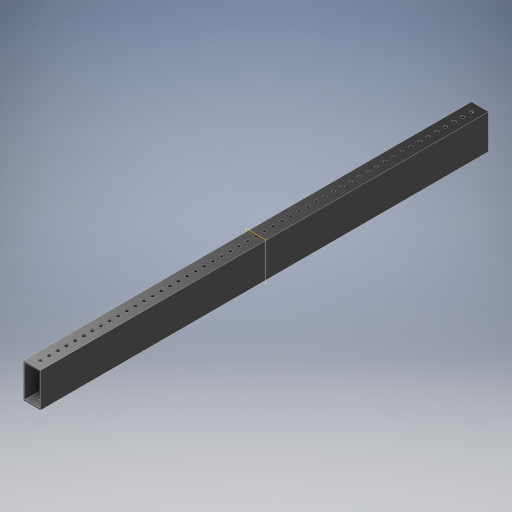
# Autodesk Inventor part: 2024-100-001-Left-Right-Extrusions
Saved by Autodesk Inventor 2024.2 (Build 282272000, 272)
## iProperties
RuleStatus: InUse
Created: 2024-01-06
Part Number: 2024-100-001-Left-Right-Extrusions
Material: Aluminum 6061
Document SubType Name: Modeling
Designer: rohan
Density: 2.7 g/cm^3
Appearance: Glossy - Black
AfterDocNew0: OnNew
AfterDocNew1: Configure
AfterAnyParamChange0: Run All Loop
AfterAnyUserParamChange0: Run All Loop
AfterFeatureSuppressionChange0: Run All Loop
PartBodyChanged0: Run All Loop
Author: rohan
Autodesk Inventor part; units mm, degrees
ref_plane "YZ Plane" through (0, 0, 0) normal (1, 0, 0) x (0, 1, 0)
sketch "Corner" plane through (0, 0, 0) normal (0, 0, 1) x (1, 0, 0)
  line L0 (-6.5971, 24.384) -> (-10.9924, 24.384)
  arc A0 (-10.9924, 24.384) -> (-11.684, 23.6924) centre (-10.9924, 23.6924) ccw
  line L1 (-11.684, 23.6924) -> (-11.684, 19.2971)
  arc A1 (-11.684, 19.2971) -> (-10.3994, 18.9412) centre (-10.9924, 19.2971) ccw
  arc A2 (-6.2412, 23.0994) -> (-6.5971, 24.384) centre (-6.5971, 23.6924) ccw
  arc A3 (-6.2412, 23.0994) -> (-10.3994, 18.9412) centre (0, 12.7) ccw
  arc A4 (-4.8895, 22.679) -> (-9.979, 17.5895) centre (0, 12.7) ccw
  line L2 (-9.979, 17.5895) -> (-11.684, 17.5895)
  line L3 (-4.8895, 22.679) -> (-4.8895, 24.384)
  line L4 (-11.684, 23.6924) -> (-11.684, 24.384)
  line L5 (-11.684, 24.384) -> (-10.9924, 24.384)
  line L6 (-11.684, 17.5895) -> (-11.684, 19.2971)
  line L7 (-4.8895, 24.384) -> (-6.5971, 24.384)
  point P0 (-8.4584, 21.1584)
  dimension "d3" = 1.5875
  dimension "d4" = 11.1125
  dimension "d8" = 0
  dimension "d9" = 0
  dimension "d10" = 0
  dimension "d11" = 2.159
  dimension "d12" = 2.159
  dimension "d5" = 1.016
  dimension "d6" = 1.705
  dimension "d7" = 0.6916
  measures "d6" distance of point (-4.889, 22.679) L7.start
  measures "d7" radius of A0
sketch "MAXTube" plane through (0, 0, 0) normal (0, 0, 1) x (1, 0, 0)
  arc A0 (-5.3052, 13.2526) -> (-8.8244, 11.2207) centre (0, 0) ccw
  arc A1 (-11.1818, 11.0863) -> (-8.8244, 11.2207) centre (-10.0994, 12.842) ccw
  arc A2 (-11.1818, 11.0863) -> (-13.8706, 10.5882) centre (-12.251, 9.3519) ccw
  arc A3 (-13.8706, 10.5882) -> (-16.1049, 6.7182) centre (0, 0) ccw
  arc A4 (-16.1049, 6.7182) -> (-15.1919, 4.1406) centre (-14.2245, 5.9338) ccw
  arc A5 (-14.1297, 2.0318) -> (-15.1919, 4.1406) centre (-16.1712, 2.3254) ccw
  arc A6 (-14.1297, 2.0318) -> (-14.1297, -2.0318) centre (0, 0) ccw
  arc A7 (-15.1919, -4.1406) -> (-14.1297, -2.0318) centre (-16.1712, -2.3254) ccw
  arc A8 (-15.1919, -4.1406) -> (-16.1049, -6.7182) centre (-14.2245, -5.9338) ccw
  arc A9 (-16.1049, -6.7182) -> (-13.8706, -10.5882) centre (0, 0) ccw
  arc A10 (-13.8706, -10.5882) -> (-11.1818, -11.0863) centre (-12.251, -9.3519) ccw
  arc A11 (-8.8244, -11.2207) -> (-11.1818, -11.0863) centre (-10.0994, -12.842) ccw
  arc A12 (-8.8244, -11.2207) -> (-5.3052, -13.2526) centre (0, 0) ccw
  arc A13 (-4.0101, -15.2268) -> (-5.3052, -13.2526) centre (-6.0718, -15.1673) ccw
  arc A14 (-4.0101, -15.2268) -> (-2.2343, -17.3064) centre (-1.9735, -15.2856) ccw
  arc A15 (-2.2343, -17.3064) -> (2.2343, -17.3064) centre (0, 0) ccw
  arc A16 (2.2343, -17.3064) -> (4.0101, -15.2268) centre (1.9735, -15.2856) ccw
  arc A17 (5.3052, -13.2526) -> (4.0101, -15.2268) centre (6.0718, -15.1673) ccw
  arc A18 (5.3052, -13.2526) -> (8.8244, -11.2207) centre (0, 0) ccw
  arc A19 (11.1818, -11.0863) -> (8.8244, -11.2207) centre (10.0994, -12.842) ccw
  arc A20 (11.1818, -11.0863) -> (13.8706, -10.5882) centre (12.251, -9.3519) ccw
  arc A21 (13.8706, -10.5882) -> (16.1049, -6.7182) centre (0, 0) ccw
  arc A22 (16.1049, -6.7182) -> (15.1919, -4.1406) centre (14.2245, -5.9338) ccw
  arc A23 (14.1297, -2.0318) -> (15.1919, -4.1406) centre (16.1712, -2.3254) ccw
  arc A24 (14.1297, -2.0318) -> (14.1297, 2.0318) centre (0, 0) ccw
  arc A25 (15.1919, 4.1406) -> (14.1297, 2.0318) centre (16.1712, 2.3254) ccw
  arc A26 (15.1919, 4.1406) -> (16.1049, 6.7182) centre (14.2245, 5.9338) ccw
  arc A27 (16.1049, 6.7182) -> (13.8706, 10.5882) centre (0, 0) ccw
  arc A28 (13.8706, 10.5882) -> (11.1818, 11.0863) centre (12.251, 9.3519) ccw
  arc A29 (8.8244, 11.2207) -> (11.1818, 11.0863) centre (10.0994, 12.842) ccw
  arc A30 (8.8244, 11.2207) -> (5.3052, 13.2526) centre (0, 0) ccw
  arc A31 (4.0101, 15.2268) -> (5.3052, 13.2526) centre (6.0718, 15.1673) ccw
  arc A32 (4.0101, 15.2268) -> (2.2343, 17.3064) centre (1.9735, 15.2856) ccw
  arc A33 (2.2343, 17.3064) -> (-2.2343, 17.3064) centre (0, 0) ccw
  arc A34 (-2.2343, 17.3064) -> (-4.0101, 15.2268) centre (-1.9735, 15.2856) ccw
  arc A35 (-5.3052, 13.2526) -> (-4.0101, 15.2268) centre (-6.0718, 15.1673) ccw
  arc A36 (-4.7199, 11.7904) -> (-7.8508, 9.9827) centre (0, 0) ccw
  arc A37 (-4.7199, 11.7904) -> (-2.4358, 15.2723) centre (-6.0718, 15.1673) ccw
  arc A38 (-2.0327, 15.7443) -> (-2.4358, 15.2723) centre (-1.9735, 15.2856) ccw
  arc A39 (2.0327, 15.7443) -> (-2.0327, 15.7443) centre (0, 0) ccw
  arc A40 (2.4358, 15.2723) -> (2.0327, 15.7443) centre (1.9735, 15.2856) ccw
  arc A41 (2.4358, 15.2723) -> (4.7199, 11.7904) centre (6.0718, 15.1673) ccw
  arc A42 (7.8508, 9.9827) -> (4.7199, 11.7904) centre (0, 0) ccw
  arc A43 (7.8508, 9.9827) -> (12.0083, 9.7456) centre (10.0994, 12.842) ccw
  arc A44 (12.6186, 9.6325) -> (12.0083, 9.7456) centre (12.251, 9.3519) ccw
  arc A45 (14.6513, 6.1118) -> (12.6186, 9.6325) centre (0, 0) ccw
  arc A46 (14.4441, 5.5267) -> (14.6513, 6.1118) centre (14.2245, 5.9338) ccw
  arc A47 (14.4441, 5.5267) -> (12.5707, 1.8076) centre (16.1712, 2.3254) ccw
  arc A48 (12.5707, -1.8076) -> (12.5707, 1.8076) centre (0, 0) ccw
  arc A49 (12.5707, -1.8076) -> (14.4441, -5.5267) centre (16.1712, -2.3254) ccw
  arc A50 (14.6513, -6.1118) -> (14.4441, -5.5267) centre (14.2245, -5.9338) ccw
  arc A51 (12.6186, -9.6325) -> (14.6513, -6.1118) centre (0, 0) ccw
  arc A52 (12.0083, -9.7456) -> (12.6186, -9.6325) centre (12.251, -9.3519) ccw
  arc A53 (12.0083, -9.7456) -> (7.8508, -9.9827) centre (10.0994, -12.842) ccw
  arc A54 (4.7199, -11.7904) -> (7.8508, -9.9827) centre (0, 0) ccw
  arc A55 (4.7199, -11.7904) -> (2.4358, -15.2723) centre (6.0718, -15.1673) ccw
  arc A56 (2.0327, -15.7443) -> (2.4358, -15.2723) centre (1.9735, -15.2856) ccw
  arc A57 (-2.0327, -15.7443) -> (2.0327, -15.7443) centre (0, 0) ccw
  arc A58 (-2.4358, -15.2723) -> (-2.0327, -15.7443) centre (-1.9735, -15.2856) ccw
  arc A59 (-2.4358, -15.2723) -> (-4.7199, -11.7904) centre (-6.0718, -15.1673) ccw
  arc A60 (-7.8508, -9.9827) -> (-4.7199, -11.7904) centre (0, 0) ccw
  arc A61 (-7.8508, -9.9827) -> (-12.0083, -9.7456) centre (-10.0994, -12.842) ccw
  arc A62 (-12.6186, -9.6325) -> (-12.0083, -9.7456) centre (-12.251, -9.3519) ccw
  arc A63 (-14.6513, -6.1118) -> (-12.6186, -9.6325) centre (0, 0) ccw
  arc A64 (-14.4441, -5.5267) -> (-14.6513, -6.1118) centre (-14.2245, -5.9338) ccw
  arc A65 (-14.4441, -5.5267) -> (-12.5707, -1.8076) centre (-16.1712, -2.3254) ccw
  arc A66 (-12.5707, 1.8076) -> (-12.5707, -1.8076) centre (0, 0) ccw
  arc A67 (-12.5707, 1.8076) -> (-14.4441, 5.5267) centre (-16.1712, 2.3254) ccw
  arc A68 (-14.6513, 6.1118) -> (-14.4441, 5.5267) centre (-14.2245, 5.9338) ccw
  arc A69 (-12.6186, 9.6325) -> (-14.6513, 6.1118) centre (0, 0) ccw
  arc A70 (-12.0083, 9.7456) -> (-12.6186, 9.6325) centre (-12.251, 9.3519) ccw
  arc A71 (-12.0083, 9.7456) -> (-7.8508, 9.9827) centre (-10.0994, 12.842) ccw
  point P0 (0, 0)
sketch "Base Sketch" plane through (0, 0, 0) normal (0, 0, 1) x (1, 0, 0)
  line L0 (-12.7, -25.4) -> (12.7, -25.4)
  line L1 (12.7, -25.4) -> (12.7, 25.4)
  line L2 (12.7, 25.4) -> (-12.7, 25.4)
  line L3 (-12.7, 25.4) -> (-12.7, -25.4)
  line L4 (-12.7, -25.4) -> (12.7, 25.4) construction
  line L5 (12.7, -25.4) -> (-12.7, 25.4) construction
  line L6 (-11.1125, -23.8125) -> (11.1125, -23.8125)
  line L7 (11.1125, -23.8125) -> (11.1125, 23.8125)
  line L8 (11.1125, 23.8125) -> (-11.1125, 23.8125)
  line L9 (-11.1125, 23.8125) -> (-11.1125, -23.8125)
  line L10 (-11.1125, -23.8125) -> (11.1125, 23.8125) construction
  line L11 (11.1125, -23.8125) -> (-11.1125, 23.8125) construction
  line L12 (-0.127, 25.4) -> (0, 25.273)
  line L13 (0, 25.273) -> (0.127, 25.4)
  line L14 (-0.127, -25.4) -> (0, -25.273)
  line L15 (0, -25.273) -> (0.127, -25.4)
  line L16 (-12.7, -12.573) -> (-12.573, -12.7)
  line L17 (-12.573, -12.7) -> (-12.7, -12.827)
  line L18 (12.7, -12.573) -> (12.573, -12.7)
  line L19 (12.7, -12.827) -> (12.573, -12.7)
  line L20 (-12.7, 12.827) -> (-12.573, 12.7)
  line L21 (-12.573, 12.7) -> (-12.7, 12.573)
  line L22 (12.7, 12.827) -> (12.573, 12.7)
  line L23 (12.573, 12.7) -> (12.7, 12.573)
  line L24 (-12.7, 0.127) -> (-12.573, 0)
  line L25 (-12.573, 0) -> (-12.7, -0.127)
  line L26 (12.7, 0.127) -> (12.573, 0)
  line L27 (12.573, 0) -> (12.7, -0.127)
  line L28 (-6.5971, 24.384) -> (-10.9924, 24.384)
  arc A0 (-10.9924, 24.384) -> (-11.684, 23.6924) centre (-10.9924, 23.6924) ccw
  line L29 (-11.684, 23.6924) -> (-11.684, 19.2971)
  arc A1 (-11.684, 19.2971) -> (-10.3994, 18.9412) centre (-10.9924, 19.2971) ccw
  arc A2 (-6.2412, 23.0994) -> (-6.5971, 24.384) centre (-6.5971, 23.6924) ccw
  arc A3 (-6.2412, 23.0994) -> (-10.3994, 18.9412) centre (0, 12.7) ccw
  arc A4 (-4.8895, 22.679) -> (-9.979, 17.5895) centre (0, 12.7) ccw
  line L30 (-9.979, 17.5895) -> (-11.684, 17.5895)
  line L31 (-4.8895, 22.679) -> (-4.8895, 24.384)
  line L32 (-11.684, 23.6924) -> (-11.684, 24.384)
  line L33 (-11.684, 24.384) -> (-10.9924, 24.384)
  line L34 (-11.684, 17.5895) -> (-11.684, 19.2971)
  line L35 (-4.8895, 24.384) -> (-6.5971, 24.384)
  line L36 (11.684, 19.2971) -> (11.684, 23.6924)
  arc A5 (11.684, 23.6924) -> (10.9924, 24.384) centre (10.9924, 23.6924) ccw
  line L37 (10.9924, 24.384) -> (6.5971, 24.384)
  arc A6 (6.5971, 24.384) -> (6.2412, 23.0994) centre (6.5971, 23.6924) ccw
  arc A7 (10.3994, 18.9412) -> (11.684, 19.2971) centre (10.9924, 19.2971) ccw
  arc A8 (10.3994, 18.9412) -> (6.2412, 23.0994) centre (0, 12.7) ccw
  arc A9 (9.979, 17.5895) -> (4.8895, 22.679) centre (0, 12.7) ccw
  line L38 (4.8895, 22.679) -> (4.8895, 24.384)
  line L39 (9.979, 17.5895) -> (11.684, 17.5895)
  line L40 (10.9924, 24.384) -> (11.684, 24.384)
  line L41 (11.684, 24.384) -> (11.684, 23.6924)
  line L42 (4.8895, 24.384) -> (6.5971, 24.384)
  line L43 (11.684, 17.5895) -> (11.684, 19.2971)
  line L44 (6.5971, -24.384) -> (10.9924, -24.384)
  arc A10 (10.9924, -24.384) -> (11.684, -23.6924) centre (10.9924, -23.6924) ccw
  line L45 (11.684, -23.6924) -> (11.684, -19.2971)
  arc A11 (11.684, -19.2971) -> (10.3994, -18.9412) centre (10.9924, -19.2971) ccw
  arc A12 (6.2412, -23.0994) -> (6.5971, -24.384) centre (6.5971, -23.6924) ccw
  arc A13 (6.2412, -23.0994) -> (10.3994, -18.9412) centre (0, -12.7) ccw
  arc A14 (4.8895, -22.679) -> (9.979, -17.5895) centre (0, -12.7) ccw
  line L46 (9.979, -17.5895) -> (11.684, -17.5895)
  line L47 (4.8895, -22.679) -> (4.8895, -24.384)
  line L48 (11.684, -23.6924) -> (11.684, -24.384)
  line L49 (11.684, -24.384) -> (10.9924, -24.384)
  line L50 (11.684, -17.5895) -> (11.684, -19.2971)
  line L51 (4.8895, -24.384) -> (6.5971, -24.384)
  line L52 (-11.684, -19.2971) -> (-11.684, -23.6924)
  arc A15 (-11.684, -23.6924) -> (-10.9924, -24.384) centre (-10.9924, -23.6924) ccw
  line L53 (-10.9924, -24.384) -> (-6.5971, -24.384)
  arc A16 (-6.5971, -24.384) -> (-6.2412, -23.0994) centre (-6.5971, -23.6924) ccw
  arc A17 (-10.3994, -18.9412) -> (-11.684, -19.2971) centre (-10.9924, -19.2971) ccw
  arc A18 (-10.3994, -18.9412) -> (-6.2412, -23.0994) centre (0, -12.7) ccw
  arc A19 (-9.979, -17.5895) -> (-4.8895, -22.679) centre (0, -12.7) ccw
  line L54 (-4.8895, -22.679) -> (-4.8895, -24.384)
  line L55 (-9.979, -17.5895) -> (-11.684, -17.5895)
  line L56 (-10.9924, -24.384) -> (-11.684, -24.384)
  line L57 (-11.684, -24.384) -> (-11.684, -23.6924)
  line L58 (-4.8895, -24.384) -> (-6.5971, -24.384)
  line L59 (-11.684, -17.5895) -> (-11.684, -19.2971)
  point P0 (0, 0)
  point P1 (-12.7, 0)
  dimension "d17" = 1.016
  dimension "d0" = 50.8
  dimension "d1" = 25.4
  dimension "d2" = 1.5875
  dimension "d3" = 1.5875
  dimension "d16" = 1.016
  dimension "d18" = 1.016
  dimension "d19" = 1.016
  dimension "d26" = 0.127
  dimension "d34" = 12.7
  dimension "d35" = 12.7
  constraints: 54 end point, 14 equal length, 10 point on line, 8 perpendicular, 7 parallel, 4 horizontal alignment, 4 midpoint, 2 horizontal, 2 vertical alignment, 1 vertical, 10 other
  measures "d0" distance of L0.end L1.end
  measures "d1" distance of L1.end L2.end
  measures "d2" distance between parallel lines of L1 L7
  measures "d3" distance between parallel lines of L2 L8
  measures "d26" distance from line of L12.end L2
  measures "d34" distance from line of L2 L20.end
  measures "d35" distance from line of L16.end L0
extrude "Base" add sketch "Base Sketch" along normal mid plane 660.4 contours L3 L17 L16 L25 L24 L21 L20 L2 L12 L13 L1 L22 L23 L26 L27 L18 L19 L0 L15 L14 | L14 L15 L0 | L3 L16 L17 | L3 L24 L25 | L19 L18 L1 | L3 L20 L21 | L27 L26 L1 | L23 L22 L1 | L2 L13 L12 | L6 A16 L53 A15 L52 A17 L9 | L6 L54 L58 A16 | A17 L59 L55 L9 | L6 A12 L51 L47 | L56 L57 A15 | L30 L34 A1 L9 | L6 L7 A11 L45 A10 L44 A12 | A1 L29 A0 L28 A2 L8 L9 | L7 L46 L50 A11 | A10 L48 L49 | A2 L35 L31 L8 | L32 L33 A0 | L7 A7 L43 L39 | L38 L42 A6 L8 | L7 L8 A6 L37 A5 L36 A7 | A5 L40 L41
extrude "MAX Corner" [suppressed]
extrude "MAX Corner Cut" [suppressed]
extrude "Scribe Lines" [suppressed]
ref_plane "Side Middle" through (0, 0, 0) normal (0, 0, 1) x (1, 0, 0)
ref_plane "Top Middle" through (0, 0, 0) normal (0, 0, 1) x (1, 0, 0)
sketch "Side Holes Sketch" plane through (12.7, -25.4, 330.2) normal (1, 0, 0) x (0, 0, -1)
  line L0 (0, 0) -> (0, 50.8) construction
  line L1 (0, 25.4) -> (660.4, 25.4) construction
  line L2 (660.4, 1.5875) -> (660.4, 49.2125) construction
  line L3 (660.4, 50.8) -> (0, 50.8) construction
  point P0 (330.2, 25.4)
  point P1 (12.7, 12.7)
  point P2 (12.7, 25.4)
  point P3 (12.7, 38.1)
  dimension "d38" = 12.7
  dimension "d61" = 12.7
  constraints: 2 end point, 2 midpoint, 2 vertical alignment, 1 horizontal alignment, 1 symmetric about line
  measures "d38" distance from line of L0 point (12.7, 12.7)
  measures "d61" distance from line of L1 point (12.7, 12.7)
hole "Top Side Hole" [suppressed]
hole "Mid Side Hole" [suppressed]
hole "Btm Side Hole" [suppressed]
pattern_linear "Side Holes" [suppressed]
mirror "Side Mirror" [suppressed]
sketch "Sketch3" plane through (12.7, -25.4, 330.2) normal (1, 0, 0) x (0, 0, -1)
  line L0 (0, 0) -> (0, 50.8) projected
  line L1 (660.4, 50.8) -> (0, 50.8) projected
  line L2 (660.4, 50.8) -> (660.4, 0) projected
  arc A0 (26.8793, 34.2244) -> (24.8474, 30.7052) centre (38.1, 25.4) ccw
  arc A1 (22.8732, 29.4101) -> (24.8474, 30.7052) centre (22.9327, 31.4718) ccw
  arc A2 (22.8732, 29.4101) -> (20.7936, 27.6343) centre (22.8144, 27.3735) ccw
  arc A3 (20.7936, 27.6343) -> (20.7936, 23.1657) centre (38.1, 25.4) ccw
  arc A4 (20.7936, 23.1657) -> (22.8732, 21.3899) centre (22.8144, 23.4265) ccw
  arc A5 (24.8474, 20.0948) -> (22.8732, 21.3899) centre (22.9327, 19.3282) ccw
  arc A6 (24.8474, 20.0948) -> (26.8793, 16.5756) centre (38.1, 25.4) ccw
  arc A7 (27.0137, 14.2182) -> (26.8793, 16.5756) centre (25.258, 15.3006) ccw
  arc A8 (27.0137, 14.2182) -> (27.5118, 11.5294) centre (28.7481, 13.149) ccw
  arc A9 (27.5118, 11.5294) -> (31.3818, 9.2951) centre (38.1, 25.4) ccw
  arc A10 (31.3818, 9.2951) -> (33.9594, 10.2081) centre (32.1662, 11.1755) ccw
  arc A11 (36.0682, 11.2703) -> (33.9594, 10.2081) centre (35.7746, 9.2288) ccw
  arc A12 (36.0682, 11.2703) -> (40.1318, 11.2703) centre (38.1, 25.4) ccw
  arc A13 (42.2406, 10.2081) -> (40.1318, 11.2703) centre (40.4254, 9.2288) ccw
  arc A14 (42.2406, 10.2081) -> (44.8182, 9.2951) centre (44.0338, 11.1755) ccw
  arc A15 (44.8182, 9.2951) -> (48.6882, 11.5294) centre (38.1, 25.4) ccw
  arc A16 (48.6882, 11.5294) -> (49.1863, 14.2182) centre (47.4519, 13.149) ccw
  arc A17 (49.3207, 16.5756) -> (49.1863, 14.2182) centre (50.942, 15.3006) ccw
  arc A18 (49.3207, 16.5756) -> (51.3526, 20.0948) centre (38.1, 25.4) ccw
  arc A19 (53.3268, 21.3899) -> (51.3526, 20.0948) centre (53.2673, 19.3282) ccw
  arc A20 (53.3268, 21.3899) -> (55.4064, 23.1657) centre (53.3856, 23.4265) ccw
  arc A21 (55.4064, 23.1657) -> (55.4064, 27.6343) centre (38.1, 25.4) ccw
  arc A22 (55.4064, 27.6343) -> (53.3268, 29.4101) centre (53.3856, 27.3735) ccw
  arc A23 (51.3526, 30.7052) -> (53.3268, 29.4101) centre (53.2673, 31.4718) ccw
  arc A24 (51.3526, 30.7052) -> (49.3207, 34.2244) centre (38.1, 25.4) ccw
  arc A25 (49.1863, 36.5818) -> (49.3207, 34.2244) centre (50.942, 35.4994) ccw
  arc A26 (49.1863, 36.5818) -> (48.6882, 39.2706) centre (47.4519, 37.651) ccw
  arc A27 (48.6882, 39.2706) -> (44.8182, 41.5049) centre (38.1, 25.4) ccw
  arc A28 (44.8182, 41.5049) -> (42.2406, 40.5919) centre (44.0338, 39.6245) ccw
  arc A29 (40.1318, 39.5297) -> (42.2406, 40.5919) centre (40.4254, 41.5712) ccw
  arc A30 (40.1318, 39.5297) -> (36.0682, 39.5297) centre (38.1, 25.4) ccw
  arc A31 (33.9594, 40.5919) -> (36.0682, 39.5297) centre (35.7746, 41.5712) ccw
  arc A32 (33.9594, 40.5919) -> (31.3818, 41.5049) centre (32.1662, 39.6245) ccw
  arc A33 (31.3818, 41.5049) -> (27.5118, 39.2706) centre (38.1, 25.4) ccw
  arc A34 (27.5118, 39.2706) -> (27.0137, 36.5818) centre (28.7481, 37.651) ccw
  arc A35 (26.8793, 34.2244) -> (27.0137, 36.5818) centre (25.258, 35.4994) ccw
  arc A36 (28.1173, 33.2508) -> (26.3096, 30.1199) centre (38.1, 25.4) ccw
  arc A37 (28.1173, 33.2508) -> (28.3544, 37.4083) centre (25.258, 35.4994) ccw
  arc A38 (28.4675, 38.0186) -> (28.3544, 37.4083) centre (28.7481, 37.651) ccw
  arc A39 (31.9882, 40.0513) -> (28.4675, 38.0186) centre (38.1, 25.4) ccw
  arc A40 (32.5733, 39.8441) -> (31.9882, 40.0513) centre (32.1662, 39.6245) ccw
  arc A41 (32.5733, 39.8441) -> (36.2924, 37.9707) centre (35.7746, 41.5712) ccw
  arc A42 (39.9076, 37.9707) -> (36.2924, 37.9707) centre (38.1, 25.4) ccw
  arc A43 (39.9076, 37.9707) -> (43.6267, 39.8441) centre (40.4254, 41.5712) ccw
  arc A44 (44.2118, 40.0513) -> (43.6267, 39.8441) centre (44.0338, 39.6245) ccw
  arc A45 (47.7325, 38.0186) -> (44.2118, 40.0513) centre (38.1, 25.4) ccw
  arc A46 (47.8456, 37.4083) -> (47.7325, 38.0186) centre (47.4519, 37.651) ccw
  arc A47 (47.8456, 37.4083) -> (48.0827, 33.2508) centre (50.942, 35.4994) ccw
  arc A48 (49.8904, 30.1199) -> (48.0827, 33.2508) centre (38.1, 25.4) ccw
  arc A49 (49.8904, 30.1199) -> (53.3723, 27.8358) centre (53.2673, 31.4718) ccw
  arc A50 (53.8443, 27.4327) -> (53.3723, 27.8358) centre (53.3856, 27.3735) ccw
  arc A51 (53.8443, 23.3673) -> (53.8443, 27.4327) centre (38.1, 25.4) ccw
  arc A52 (53.3723, 22.9642) -> (53.8443, 23.3673) centre (53.3856, 23.4265) ccw
  arc A53 (53.3723, 22.9642) -> (49.8904, 20.6801) centre (53.2673, 19.3282) ccw
  arc A54 (48.0827, 17.5492) -> (49.8904, 20.6801) centre (38.1, 25.4) ccw
  arc A55 (48.0827, 17.5492) -> (47.8456, 13.3917) centre (50.942, 15.3006) ccw
  arc A56 (47.7325, 12.7814) -> (47.8456, 13.3917) centre (47.4519, 13.149) ccw
  arc A57 (44.2118, 10.7487) -> (47.7325, 12.7814) centre (38.1, 25.4) ccw
  arc A58 (43.6267, 10.9559) -> (44.2118, 10.7487) centre (44.0338, 11.1755) ccw
  arc A59 (43.6267, 10.9559) -> (39.9076, 12.8293) centre (40.4254, 9.2288) ccw
  arc A60 (36.2924, 12.8293) -> (39.9076, 12.8293) centre (38.1, 25.4) ccw
  arc A61 (36.2924, 12.8293) -> (32.5733, 10.9559) centre (35.7746, 9.2288) ccw
  arc A62 (31.9882, 10.7487) -> (32.5733, 10.9559) centre (32.1662, 11.1755) ccw
  arc A63 (28.4675, 12.7814) -> (31.9882, 10.7487) centre (38.1, 25.4) ccw
  arc A64 (28.3544, 13.3917) -> (28.4675, 12.7814) centre (28.7481, 13.149) ccw
  arc A65 (28.3544, 13.3917) -> (28.1173, 17.5492) centre (25.258, 15.3006) ccw
  arc A66 (26.3096, 20.6801) -> (28.1173, 17.5492) centre (38.1, 25.4) ccw
  arc A67 (26.3096, 20.6801) -> (22.8277, 22.9642) centre (22.9327, 19.3282) ccw
  arc A68 (22.3557, 23.3673) -> (22.8277, 22.9642) centre (22.8144, 23.4265) ccw
  arc A69 (22.3557, 27.4327) -> (22.3557, 23.3673) centre (38.1, 25.4) ccw
  arc A70 (22.8277, 27.8358) -> (22.3557, 27.4327) centre (22.8144, 27.3735) ccw
  arc A71 (22.8277, 27.8358) -> (26.3096, 30.1199) centre (22.9327, 31.4718) ccw
  arc A72 (-23.9207, 34.2244) -> (-25.9526, 30.7052) centre (-12.7, 25.4) ccw
  arc A73 (-27.9268, 29.4101) -> (-25.9526, 30.7052) centre (-27.8673, 31.4718) ccw
  arc A74 (-27.9268, 29.4101) -> (-30.0064, 27.6343) centre (-27.9856, 27.3735) ccw
  arc A75 (-30.0064, 27.6343) -> (-30.0064, 23.1657) centre (-12.7, 25.4) ccw
  arc A76 (-30.0064, 23.1657) -> (-27.9268, 21.3899) centre (-27.9856, 23.4265) ccw
  arc A77 (-25.9526, 20.0948) -> (-27.9268, 21.3899) centre (-27.8673, 19.3282) ccw
  arc A78 (-25.9526, 20.0948) -> (-23.9207, 16.5756) centre (-12.7, 25.4) ccw
  arc A79 (-23.7863, 14.2182) -> (-23.9207, 16.5756) centre (-25.542, 15.3006) ccw
  arc A80 (-23.7863, 14.2182) -> (-23.2882, 11.5294) centre (-22.0519, 13.149) ccw
  arc A81 (-23.2882, 11.5294) -> (-19.4182, 9.2951) centre (-12.7, 25.4) ccw
  arc A82 (-19.4182, 9.2951) -> (-16.8406, 10.2081) centre (-18.6338, 11.1755) ccw
  arc A83 (-14.7318, 11.2703) -> (-16.8406, 10.2081) centre (-15.0254, 9.2288) ccw
  arc A84 (-14.7318, 11.2703) -> (-10.6682, 11.2703) centre (-12.7, 25.4) ccw
  arc A85 (-8.5594, 10.2081) -> (-10.6682, 11.2703) centre (-10.3746, 9.2288) ccw
  arc A86 (-8.5594, 10.2081) -> (-5.9818, 9.2951) centre (-6.7662, 11.1755) ccw
  arc A87 (-5.9818, 9.2951) -> (-2.1118, 11.5294) centre (-12.7, 25.4) ccw
  arc A88 (-2.1118, 11.5294) -> (-1.6137, 14.2182) centre (-3.3481, 13.149) ccw
  arc A89 (-1.4793, 16.5756) -> (-1.6137, 14.2182) centre (0.142, 15.3006) ccw
  arc A90 (-1.4793, 16.5756) -> (0.5526, 20.0948) centre (-12.7, 25.4) ccw
  arc A91 (2.5268, 21.3899) -> (0.5526, 20.0948) centre (2.4673, 19.3282) ccw
  arc A92 (2.5268, 21.3899) -> (4.6064, 23.1657) centre (2.5856, 23.4265) ccw
  arc A93 (4.6064, 23.1657) -> (4.6064, 27.6343) centre (-12.7, 25.4) ccw
  arc A94 (4.6064, 27.6343) -> (2.5268, 29.4101) centre (2.5856, 27.3735) ccw
  arc A95 (0.5526, 30.7052) -> (2.5268, 29.4101) centre (2.4673, 31.4718) ccw
  arc A96 (0.5526, 30.7052) -> (-1.4793, 34.2244) centre (-12.7, 25.4) ccw
  arc A97 (-1.6137, 36.5818) -> (-1.4793, 34.2244) centre (0.142, 35.4994) ccw
  arc A98 (-1.6137, 36.5818) -> (-2.1118, 39.2706) centre (-3.3481, 37.651) ccw
  arc A99 (-2.1118, 39.2706) -> (-5.9818, 41.5049) centre (-12.7, 25.4) ccw
  arc A100 (-5.9818, 41.5049) -> (-8.5594, 40.5919) centre (-6.7662, 39.6245) ccw
  arc A101 (-10.6682, 39.5297) -> (-8.5594, 40.5919) centre (-10.3746, 41.5712) ccw
  arc A102 (-10.6682, 39.5297) -> (-14.7318, 39.5297) centre (-12.7, 25.4) ccw
  arc A103 (-16.8406, 40.5919) -> (-14.7318, 39.5297) centre (-15.0254, 41.5712) ccw
  arc A104 (-16.8406, 40.5919) -> (-19.4182, 41.5049) centre (-18.6338, 39.6245) ccw
  arc A105 (-19.4182, 41.5049) -> (-23.2882, 39.2706) centre (-12.7, 25.4) ccw
  arc A106 (-23.2882, 39.2706) -> (-23.7863, 36.5818) centre (-22.0519, 37.651) ccw
  arc A107 (-23.9207, 34.2244) -> (-23.7863, 36.5818) centre (-25.542, 35.4994) ccw
  arc A108 (-22.6827, 33.2508) -> (-24.4904, 30.1199) centre (-12.7, 25.4) ccw
  arc A109 (-22.6827, 33.2508) -> (-22.4456, 37.4083) centre (-25.542, 35.4994) ccw
  arc A110 (-22.3325, 38.0186) -> (-22.4456, 37.4083) centre (-22.0519, 37.651) ccw
  arc A111 (-18.8118, 40.0513) -> (-22.3325, 38.0186) centre (-12.7, 25.4) ccw
  arc A112 (-18.2267, 39.8441) -> (-18.8118, 40.0513) centre (-18.6338, 39.6245) ccw
  arc A113 (-18.2267, 39.8441) -> (-14.5076, 37.9707) centre (-15.0254, 41.5712) ccw
  arc A114 (-10.8924, 37.9707) -> (-14.5076, 37.9707) centre (-12.7, 25.4) ccw
  arc A115 (-10.8924, 37.9707) -> (-7.1733, 39.8441) centre (-10.3746, 41.5712) ccw
  arc A116 (-6.5882, 40.0513) -> (-7.1733, 39.8441) centre (-6.7662, 39.6245) ccw
  arc A117 (-3.0675, 38.0186) -> (-6.5882, 40.0513) centre (-12.7, 25.4) ccw
  arc A118 (-2.9544, 37.4083) -> (-3.0675, 38.0186) centre (-3.3481, 37.651) ccw
  arc A119 (-2.9544, 37.4083) -> (-2.7173, 33.2508) centre (0.142, 35.4994) ccw
  arc A120 (-0.9096, 30.1199) -> (-2.7173, 33.2508) centre (-12.7, 25.4) ccw
  arc A121 (-0.9096, 30.1199) -> (2.5723, 27.8358) centre (2.4673, 31.4718) ccw
  arc A122 (3.0443, 27.4327) -> (2.5723, 27.8358) centre (2.5856, 27.3735) ccw
  arc A123 (3.0443, 23.3673) -> (3.0443, 27.4327) centre (-12.7, 25.4) ccw
  arc A124 (2.5723, 22.9642) -> (3.0443, 23.3673) centre (2.5856, 23.4265) ccw
  arc A125 (2.5723, 22.9642) -> (-0.9096, 20.6801) centre (2.4673, 19.3282) ccw
  arc A126 (-2.7173, 17.5492) -> (-0.9096, 20.6801) centre (-12.7, 25.4) ccw
  arc A127 (-2.7173, 17.5492) -> (-2.9544, 13.3917) centre (0.142, 15.3006) ccw
  arc A128 (-3.0675, 12.7814) -> (-2.9544, 13.3917) centre (-3.3481, 13.149) ccw
  arc A129 (-6.5882, 10.7487) -> (-3.0675, 12.7814) centre (-12.7, 25.4) ccw
  arc A130 (-7.1733, 10.9559) -> (-6.5882, 10.7487) centre (-6.7662, 11.1755) ccw
  arc A131 (-7.1733, 10.9559) -> (-10.8924, 12.8293) centre (-10.3746, 9.2288) ccw
  arc A132 (-14.5076, 12.8293) -> (-10.8924, 12.8293) centre (-12.7, 25.4) ccw
  arc A133 (-14.5076, 12.8293) -> (-18.2267, 10.9559) centre (-15.0254, 9.2288) ccw
  arc A134 (-18.8118, 10.7487) -> (-18.2267, 10.9559) centre (-18.6338, 11.1755) ccw
  arc A135 (-22.3325, 12.7814) -> (-18.8118, 10.7487) centre (-12.7, 25.4) ccw
  arc A136 (-22.4456, 13.3917) -> (-22.3325, 12.7814) centre (-22.0519, 13.149) ccw
  arc A137 (-22.4456, 13.3917) -> (-22.6827, 17.5492) centre (-25.542, 15.3006) ccw
  arc A138 (-24.4904, 20.6801) -> (-22.6827, 17.5492) centre (-12.7, 25.4) ccw
  arc A139 (-24.4904, 20.6801) -> (-27.9723, 22.9642) centre (-27.8673, 19.3282) ccw
  arc A140 (-28.4443, 23.3673) -> (-27.9723, 22.9642) centre (-27.9856, 23.4265) ccw
  arc A141 (-28.4443, 27.4327) -> (-28.4443, 23.3673) centre (-12.7, 25.4) ccw
  arc A142 (-27.9723, 27.8358) -> (-28.4443, 27.4327) centre (-27.9856, 27.3735) ccw
  arc A143 (-27.9723, 27.8358) -> (-24.4904, 30.1199) centre (-27.8673, 31.4718) ccw
  arc A144 (636.4793, 34.2244) -> (634.4474, 30.7052) centre (647.7, 25.4) ccw
  arc A145 (632.4732, 29.4101) -> (634.4474, 30.7052) centre (632.5327, 31.4718) ccw
  arc A146 (632.4732, 29.4101) -> (630.3936, 27.6343) centre (632.4144, 27.3735) ccw
  arc A147 (630.3936, 27.6343) -> (630.3936, 23.1657) centre (647.7, 25.4) ccw
  arc A148 (630.3936, 23.1657) -> (632.4732, 21.3899) centre (632.4144, 23.4265) ccw
  arc A149 (634.4474, 20.0948) -> (632.4732, 21.3899) centre (632.5327, 19.3282) ccw
  arc A150 (634.4474, 20.0948) -> (636.4793, 16.5756) centre (647.7, 25.4) ccw
  arc A151 (636.6137, 14.2182) -> (636.4793, 16.5756) centre (634.858, 15.3006) ccw
  arc A152 (636.6137, 14.2182) -> (637.1118, 11.5294) centre (638.3481, 13.149) ccw
  arc A153 (637.1118, 11.5294) -> (640.9818, 9.2951) centre (647.7, 25.4) ccw
  arc A154 (640.9818, 9.2951) -> (643.5594, 10.2081) centre (641.7662, 11.1755) ccw
  arc A155 (645.6682, 11.2703) -> (643.5594, 10.2081) centre (645.3746, 9.2288) ccw
  arc A156 (645.6682, 11.2703) -> (649.7318, 11.2703) centre (647.7, 25.4) ccw
  arc A157 (651.8406, 10.2081) -> (649.7318, 11.2703) centre (650.0254, 9.2288) ccw
  arc A158 (651.8406, 10.2081) -> (654.4182, 9.2951) centre (653.6338, 11.1755) ccw
  arc A159 (654.4182, 9.2951) -> (658.2882, 11.5294) centre (647.7, 25.4) ccw
  arc A160 (658.2882, 11.5294) -> (658.7863, 14.2182) centre (657.0519, 13.149) ccw
  arc A161 (658.9207, 16.5756) -> (658.7863, 14.2182) centre (660.542, 15.3006) ccw
  arc A162 (658.9207, 16.5756) -> (660.9526, 20.0948) centre (647.7, 25.4) ccw
  arc A163 (662.9268, 21.3899) -> (660.9526, 20.0948) centre (662.8673, 19.3282) ccw
  arc A164 (662.9268, 21.3899) -> (665.0064, 23.1657) centre (662.9856, 23.4265) ccw
  arc A165 (665.0064, 23.1657) -> (665.0064, 27.6343) centre (647.7, 25.4) ccw
  arc A166 (665.0064, 27.6343) -> (662.9268, 29.4101) centre (662.9856, 27.3735) ccw
  arc A167 (660.9526, 30.7052) -> (662.9268, 29.4101) centre (662.8673, 31.4718) ccw
  arc A168 (660.9526, 30.7052) -> (658.9207, 34.2244) centre (647.7, 25.4) ccw
  arc A169 (658.7863, 36.5818) -> (658.9207, 34.2244) centre (660.542, 35.4994) ccw
  arc A170 (658.7863, 36.5818) -> (658.2882, 39.2706) centre (657.0519, 37.651) ccw
  arc A171 (658.2882, 39.2706) -> (654.4182, 41.5049) centre (647.7, 25.4) ccw
  arc A172 (654.4182, 41.5049) -> (651.8406, 40.5919) centre (653.6338, 39.6245) ccw
  arc A173 (649.7318, 39.5297) -> (651.8406, 40.5919) centre (650.0254, 41.5712) ccw
  arc A174 (649.7318, 39.5297) -> (645.6682, 39.5297) centre (647.7, 25.4) ccw
  arc A175 (643.5594, 40.5919) -> (645.6682, 39.5297) centre (645.3746, 41.5712) ccw
  arc A176 (643.5594, 40.5919) -> (640.9818, 41.5049) centre (641.7662, 39.6245) ccw
  arc A177 (640.9818, 41.5049) -> (637.1118, 39.2706) centre (647.7, 25.4) ccw
  arc A178 (637.1118, 39.2706) -> (636.6137, 36.5818) centre (638.3481, 37.651) ccw
  arc A179 (636.4793, 34.2244) -> (636.6137, 36.5818) centre (634.858, 35.4994) ccw
  arc A180 (637.7173, 33.2508) -> (635.9096, 30.1199) centre (647.7, 25.4) ccw
  arc A181 (637.7173, 33.2508) -> (637.9544, 37.4083) centre (634.858, 35.4994) ccw
  arc A182 (638.0675, 38.0186) -> (637.9544, 37.4083) centre (638.3481, 37.651) ccw
  arc A183 (641.5882, 40.0513) -> (638.0675, 38.0186) centre (647.7, 25.4) ccw
  arc A184 (642.1733, 39.8441) -> (641.5882, 40.0513) centre (641.7662, 39.6245) ccw
  arc A185 (642.1733, 39.8441) -> (645.8924, 37.9707) centre (645.3746, 41.5712) ccw
  arc A186 (649.5076, 37.9707) -> (645.8924, 37.9707) centre (647.7, 25.4) ccw
  arc A187 (649.5076, 37.9707) -> (653.2267, 39.8441) centre (650.0254, 41.5712) ccw
  arc A188 (653.8118, 40.0513) -> (653.2267, 39.8441) centre (653.6338, 39.6245) ccw
  arc A189 (657.3325, 38.0186) -> (653.8118, 40.0513) centre (647.7, 25.4) ccw
  arc A190 (657.4456, 37.4083) -> (657.3325, 38.0186) centre (657.0519, 37.651) ccw
  arc A191 (657.4456, 37.4083) -> (657.6827, 33.2508) centre (660.542, 35.4994) ccw
  arc A192 (659.4904, 30.1199) -> (657.6827, 33.2508) centre (647.7, 25.4) ccw
  arc A193 (659.4904, 30.1199) -> (662.9723, 27.8358) centre (662.8673, 31.4718) ccw
  arc A194 (663.4443, 27.4327) -> (662.9723, 27.8358) centre (662.9856, 27.3735) ccw
  arc A195 (663.4443, 23.3673) -> (663.4443, 27.4327) centre (647.7, 25.4) ccw
  arc A196 (662.9723, 22.9642) -> (663.4443, 23.3673) centre (662.9856, 23.4265) ccw
  arc A197 (662.9723, 22.9642) -> (659.4904, 20.6801) centre (662.8673, 19.3282) ccw
  arc A198 (657.6827, 17.5492) -> (659.4904, 20.6801) centre (647.7, 25.4) ccw
  arc A199 (657.6827, 17.5492) -> (657.4456, 13.3917) centre (660.542, 15.3006) ccw
  arc A200 (657.3325, 12.7814) -> (657.4456, 13.3917) centre (657.0519, 13.149) ccw
  arc A201 (653.8118, 10.7487) -> (657.3325, 12.7814) centre (647.7, 25.4) ccw
  arc A202 (653.2267, 10.9559) -> (653.8118, 10.7487) centre (653.6338, 11.1755) ccw
  arc A203 (653.2267, 10.9559) -> (649.5076, 12.8293) centre (650.0254, 9.2288) ccw
  arc A204 (645.8924, 12.8293) -> (649.5076, 12.8293) centre (647.7, 25.4) ccw
  arc A205 (645.8924, 12.8293) -> (642.1733, 10.9559) centre (645.3746, 9.2288) ccw
  arc A206 (641.5882, 10.7487) -> (642.1733, 10.9559) centre (641.7662, 11.1755) ccw
  arc A207 (638.0675, 12.7814) -> (641.5882, 10.7487) centre (647.7, 25.4) ccw
  arc A208 (637.9544, 13.3917) -> (638.0675, 12.7814) centre (638.3481, 13.149) ccw
  arc A209 (637.9544, 13.3917) -> (637.7173, 17.5492) centre (634.858, 15.3006) ccw
  arc A210 (635.9096, 20.6801) -> (637.7173, 17.5492) centre (647.7, 25.4) ccw
  arc A211 (635.9096, 20.6801) -> (632.4277, 22.9642) centre (632.5327, 19.3282) ccw
  arc A212 (631.9557, 23.3673) -> (632.4277, 22.9642) centre (632.4144, 23.4265) ccw
  arc A213 (631.9557, 27.4327) -> (631.9557, 23.3673) centre (647.7, 25.4) ccw
  arc A214 (632.4277, 27.8358) -> (631.9557, 27.4327) centre (632.4144, 27.3735) ccw
  arc A215 (632.4277, 27.8358) -> (635.9096, 30.1199) centre (632.5327, 31.4718) ccw
  point P0 (330.2, 25.4)
  point P1 (0, 25.4)
  point P2 (30.1625, 39.1482)
  point P3 (46.0375, 11.6518)
  point P4 (30.1625, 39.1482)
  point P5 (0, 28.8128)
  point P6 (0, 25.4)
  point P7 (0, 28.799)
  point P8 (569.0108, 12.7)
  point P9 (660.4, 31.9181)
  point P10 (660.4, 18.8819)
  dimension "d78" = 50.8
  dimension "d98" = 609.6
  dimension "d69" = 38.1
  dimension "d93" = 25.4
  dimension "d97" = 12.7
  constraints: 1 midpoint, 3 other
extrude "MAXTube Hole" [suppressed]
extrude "MAXTube Outside" [suppressed]
pattern_linear "MAXTube Pattern" [suppressed]
mirror "MAXTube Mirror" [suppressed]
sketch "Sketch4" plane through (-12.7, 25.4, 330.2) normal (0, 1, 0) x (1, 0, 0)
  circle A0 centre (12.7, 12.7) radius 2.4892
  circle A1 centre (12.7, 12.7) radius 2.4892
  circle A2 centre (12.7, 12.7) radius 2.4892
  line L0 (25.4, 0) -> (0, 0) projected
  point P0 (12.7, 330.2)
  point P1 (12.573, 0)
  dimension "d80" = 4.9784
  dimension "d81" = 0
  dimension "d82" = 0
  dimension "d83" = 12.7
  constraints: 3 centre point, 2 coincident, 2 concentric, 1 vertical alignment
  measures "d80" diameter of A0
  measures "d81" distance of A1.centre A0.centre
  measures "d82" distance of A1.centre A2.centre
  measures "d83" distance from line of L0 A0.centre
extrude "Left Top Hole" cut sketch "Sketch4" against normal through all
extrude "Mid Top Hole" [suppressed]
extrude "Right Top Hole" [suppressed]
pattern_linear "Top Holes" count 26 spacing 12.7 along (0, 0, -1) of "Left Top Hole"
mirror "Top Mirror" about plane through (0, 0, 0) normal (0, 0, 1) of "Left Top Hole", "Top Holes"
sketch "Sketch5" plane through (-12.7, -25.4, 330.2) normal (0, -1, 0) x (1, 0, 0)
  circle A0 centre (12.7, -38.1) radius 2.4892 projected
  circle A1 centre (12.7, -63.5) radius 2.4892 projected
  circle A2 centre (12.7, -88.9) radius 2.4892 projected
  circle A3 centre (12.7, -114.3) radius 2.4892 projected
  circle A4 centre (12.7, -609.6) radius 2.4892 projected
  circle A5 centre (12.7, -584.2) radius 2.4892 projected
  circle A6 centre (12.7, -558.8) radius 2.4892 projected
  circle A7 centre (12.7, -533.4) radius 2.4892 projected
  circle A8 centre (12.7, -38.1) radius 3.175
  circle A9 centre (12.7, -63.5) radius 3.175
  circle A10 centre (12.7, -88.9) radius 3.175
  circle A11 centre (12.7, -114.3) radius 3.175
  line L0 (25.4, 0) -> (25.4, -660.4) projected
  line L1 (25.4, -330.2) -> (0, -330.2)
  line L2 (0, -660.4) -> (0, 0) projected
  circle A12 centre (12.7, -622.3) radius 3.175
  circle A13 centre (12.7, -596.9) radius 3.175
  circle A14 centre (12.7, -571.5) radius 3.175
  circle A15 centre (12.7, -546.1) radius 3.175
  point P0 (12.7, -330.2)
  dimension "d101" = 6.35
  dimension "d102" = 6.35
  dimension "d103" = 6.35
  dimension "d104" = 6.35
  constraints: 8 centre point, 4 coincident, 4 symmetric about line, 2 end point, 2 midpoint, 4 other
  measures "d101" diameter of A8
  measures "d102" diameter of A9
  measures "d103" diameter of A10
  measures "d104" diameter of A11
extrude "Extrusion11" cut sketch "Sketch5" against normal blind 12.7 contours A8 | A9 | A10 | A11 | A12 | A13 | A14 | A15
ref_plane "Work Plane5" through (0, 0, 0) normal (0, 0, 1) x (1, 0, 0)
ref_plane "Work Plane3" through (0, 0, -18.2563) normal (0, 0, 1) x (1, 0, 0)
equation "\"d3\" = WidthWall"
equation "\"d61\" = SideMiddleSpace"
equation "\"d12\" = d11"
equation "\"d0\" = Height"
equation "\"d1\" = Width"
equation "\"d2\" = HeightWall"
equation "\"d20\" = Length"
equation "\"d22\" = Length"
equation "\"Height\" = 50.8"
equation "\"Width\" = 25.4"
equation "\"HeightWall\" = 1.5875"
equation "\"WidthWall\" = 1.5875"
equation "\"Length\" = 660.4"
equation "\"Wall\" = 1.5875"
equation "\"PlaneOffset_Side\" = -330.2"
equation "\"SideMiddleSpace\" = 12.7"
equation "\"Side_Length_Edge\" = 12.7"
equation "\"Side_Width_Space\" = 12.7"
equation "\"Side_Length_Space\" = 50.8"
equation "\"Side_Width_Count\" = 0"
equation "\"Side_Width_Edge\" = 12.7"
equation "\"Top_Width_Edge\" = 12.7"
equation "\"Top_Width_Space\" = 6.35"
equation "\"Top_Length_Space\" = 12.7"
equation "\"Top_Length_Edge\" = 12.7"
equation "\"TopMiddleSpace\" = 0"
equation "\"PlaneOffset_Top\" = -330.2"
equation "\"HoleSize\" = 4.9784"
body "Solid1"
